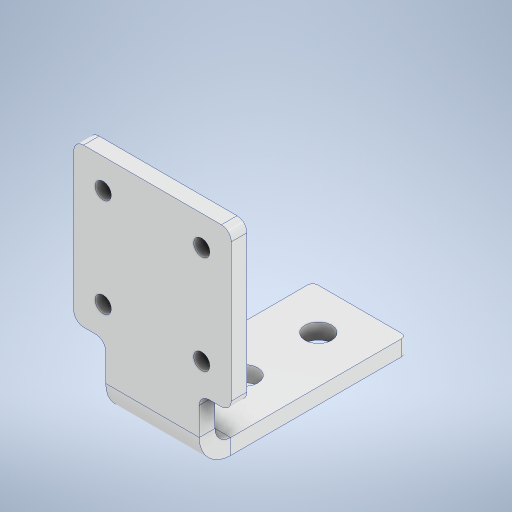
# Autodesk Inventor part: Printhead Belt Retainer Bracket
Saved by Autodesk Inventor 2024 (Build 280153000, 153)
## iProperties
Created: 2024-12-29
Part Number: Printhead Belt Retainer Bracket
Material: Aluminum 6061
Document SubType Name: Sheet Metal
Designer: Ishaan
Density: 2.7 g/cm^3
Sheet Metal Rule: SendCutSend_1-8_Alu
Appearance: Aluminum - Flat
Author: Ishaan
Autodesk Inventor part; units mm, degrees
ref_plane "YZ Plane" through (0, 0, 0) normal (1, 0, 0) x (0, 1, 0)
ref_plane "XZ Plane" through (0, 0, 0) normal (0, 1, 0) x (-1, 0, 0)
ref_plane "XY Plane" through (0, 0, 0) normal (0, 0, 1) x (1, 0, 0)
sketch "Sketch1" plane through (0, 0, 0) normal (0, 0, 1) x (1, 0, 0)
  line L0 (16, -16) -> (-16, -16)
  line L1 (-16, -16) -> (-16, 16)
  line L2 (-16, 16) -> (16, 16)
  line L3 (16, 16) -> (16, -16)
  line L4 (16, -16) -> (-16, 16) construction
  line L5 (-16, -16) -> (16, 16) construction
  line L6 (10, -10) -> (-10, -10) construction
  line L7 (-10, -10) -> (-10, 10) construction
  line L8 (-10, 10) -> (10, 10) construction
  line L9 (10, 10) -> (10, -10) construction
  line L10 (10, -10) -> (-10, 10) construction
  line L11 (-10, -10) -> (10, 10) construction
  line L12 (-9.5, -16) -> (9.5, -16)
  line L13 (9.5, -16) -> (9.5, -30)
  line L14 (9.5, -30) -> (-9.5, -30)
  line L15 (-9.5, -30) -> (-9.5, -16)
  point P0 (0, 0)
  point P1 (0, -16)
  dimension "d0" = 32
  dimension "d1" = 32
  dimension "d2" = 20
  dimension "d3" = 20
  dimension "d4" = 19
  dimension "d5" = 30
  constraints: 32 end point, 6 midpoint, 6 parallel, 3 horizontal, 3 perpendicular, 1 point on line
  measures "d0" distance of L1.end L2.end
  measures "d1" distance of L0.end L1.end
  measures "d2" distance of L7.end L8.end
  measures "d3" distance of L6.end L7.end
  measures "d4" distance of L13.end L14.end
  measures "d5" distance from line of point (0, 0) L14
extrude "Plate1" add sketch "Sketch1" along normal blind 3.175
sketch "Sketch2" plane through (-9.5, -26.825, 3.175) normal (0, -1, 0) x (1, 0, 0)
  line L0 (19, 0) -> (0, 0)
  line L1 (0, 0) -> (0, -50)
  line L2 (0, -50) -> (19, -50)
  line L3 (19, -50) -> (19, 0)
  constraints: 6 end point, 1 horizontal, 1 perpendicular, 1 vertical
edge flange "Flange1" height 50 angle 90 thickness 3.175 bend radius 3.175 thickness toward (0, -1, 0) relief tear relief width 3.175 relief depth 1.5875 edges at (0, -30, 0) wall of the first edge with corners at (9.5, -26.825, 3.175) (-9.5, -26.825, 3.175) (-9.5, -26.825, -46.825) (9.5, -26.825, -46.825)
bend "Bend1"
corner "Corner1"
fillet "Fillet1" radius 2 6 edges at (-16, -16, 1.5875) (-16, 16, 1.5875) (16, 16, 1.5875) (16, -16, 1.5875) (9.5, -16, 1.5875) (-9.5, -16, 1.5875)
hole "Hole1" at (10, -10, 0) at (10, 10, 0) at (-10, 10, 0) at (-10, -10, 0) direction (0, 0, 1) diameter 3.3 end through all
sketch "Sketch3" plane through (-9.5, -30, -46.825) normal (0, -1, 0) x (1, 0, 0)
  line L0 (1.15, 46.825) -> (-2.15, 46.825) construction
  line L1 (1.15, 46.825) -> (-2.15, 46.825) construction
  line L2 (21.15, 46.825) -> (17.85, 46.825) construction
  line L3 (21.15, 46.825) -> (17.85, 46.825) construction
  line L4 (23.5, 46.825) -> (25.5, 46.825) construction
  line L5 (21, 46.825) -> (23.5, 46.825) construction
  line L6 (19, 46.825) -> (21, 46.825) construction
  line L7 (19, 46.825) -> (0, 46.825) construction
  line L8 (-2, 46.825) -> (0, 46.825) construction
  line L9 (-4.5, 46.825) -> (-2, 46.825) construction
  line L10 (-6.5, 46.825) -> (-4.5, 46.825) construction
  line L11 (-4.5, 46.825) -> (-6.5, 46.825) construction
  line L12 (23.5, 46.825) -> (-4.5, 46.825) construction
  line L13 (25.5, 46.825) -> (23.5, 46.825) construction
  line L14 (0, 0) -> (0, 43.65) construction
  line L15 (19, 24.975) -> (0, 24.975) construction
  line L16 (0, 24.975) -> (0, 37.675) construction
  line L17 (0, 37.675) -> (19, 37.675) construction
  line L18 (19, 37.675) -> (19, 24.975) construction
  line L19 (19, 24.975) -> (0, 37.675) construction
  line L20 (0, 24.975) -> (19, 37.675) construction
  line L21 (19, 43.65) -> (19, 0) construction
  line L22 (0, 33.825) -> (19, 33.825) construction
  line L23 (19, 33.825) -> (19, 13.825) construction
  line L24 (19, 13.825) -> (0, 13.825) construction
  line L25 (0, 13.825) -> (0, 33.825) construction
  line L26 (19, 9.975) -> (0, 9.975) construction
  line L27 (0, 9.975) -> (0, 22.675) construction
  line L28 (0, 22.675) -> (19, 22.675) construction
  line L29 (19, 22.675) -> (19, 9.975) construction
  line L30 (19, 9.975) -> (0, 22.675) construction
  line L31 (0, 9.975) -> (19, 22.675) construction
  line L32 (0, 33.825) -> (19, 13.825) construction
  line L33 (0, 13.825) -> (19, 33.825) construction
  line L34 (19, 43.65) -> (0, 43.65) projected
  line L35 (0, 0) -> (0, 43.65) projected
  line L36 (19, 0) -> (0, 0) projected
  line L37 (19, 43.65) -> (19, 0) projected
  line L38 (0, 7.975) -> (19, 7.975)
  point P0 (9.5, 46.825)
  point P1 (9.5, 31.325)
  point P2 (9.5, 46.825)
  point P3 (9.5, 16.325)
  point P4 (9.5, 23.825)
  point P5 (9.5, 23.825)
  point P6 (19, 9.975)
  point P7 (0, 9.975)
  dimension "d25" = 12.7
  dimension "d27" = 20
  dimension "d28" = 13
  dimension "d29" = 7.5
  dimension "d30" = 7.5
  dimension "d33" = 2
  constraints: 38 end point, 7 midpoint, 7 parallel, 7 point on line, 4 perpendicular, 3 horizontal, 1 collinear
  measures "d25" distance of L15.end L16.end
  measures "d27" distance of L22.end L23.end
  measures "d28" distance between parallel lines of L7 L22
  measures "d29" distance of point (9.5, 31.325) point (9.5, 23.825)
  measures "d30" distance of point (9.5, 16.325) point (9.5, 23.825)
  measures "d33" distance between parallel lines of L26 L38
extrude "Extrusion1" cut sketch "Sketch3" against normal through all contours L37 L36 L35 L38
fillet "Fillet2" radius 1 2 edges at (9.5, -28.4125, -38.85) (-9.5, -28.4125, -38.85)
hole "Hole2" at (0, -30, -15.5) at (0, -30, -30.5) direction (0, 1, 0) diameter 5.4 end through all
equation "\"d23\" = Thickness"
equation "\"d6\" = Thickness"
equation "\"d7\" = BendReliefWidth"
equation "\"d8\" = BendReliefDepth"
equation "\"d9\" = MinimumRemnant"
equation "\"d10\" = TransitionRadius"
equation "\"d13\" = BendRadius"
equation "\"d14\" = CornerReliefSize"
equation "\"d15\" = GapSize"
equation "\"d16\" = JacobiRadiusSize"
equation "\"d30\" = d29"
equation "\"BendReliefWidth\" = Thickness"
equation "\"BendReliefDepth\" = 0.5 * Thickness"
equation "\"CornerReliefSize\" = 4 * Thickness"
equation "\"MinimumRemnant\" = 2 * Thickness"
equation "\"TransitionRadius\" = BendRadius"
equation "\"JacobiRadiusSize\" = BendRadius"
equation "\"GapSize\" = Thickness"
equation "\"Thickness\" = 3.175"
equation "\"BendRadius\" = 3.175"
body "Solid1"
